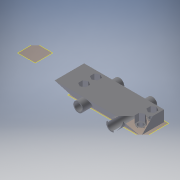
# Autodesk Inventor part: 23_Connection_Smartphone
Saved by Autodesk Inventor 2016 (Build 200138000, 138)
## iProperties
Created: 2016-10-24
Part Number: 23_Connection_Smartphone
Material: Generisch
Document SubType Name: Modeling
Designer: Bene
Density: 1 g/cm^3
Appearance: Vorgabe
Author: Bene
Autodesk Inventor part; units mm, degrees
ref_plane "YZ Plane" through (0, 0, 0) normal (1, 0, 0) x (0, 1, 0)
ref_plane "XZ Plane" through (0, 0, 0) normal (0, 1, 0) x (-1, 0, 0)
ref_plane "XY Plane" through (0, 0, 0) normal (0, 0, 1) x (1, 0, 0)
ref_plane "Arbeitsebene1" through (0, 0, 0) normal (0, 0, 1) x (1, 0, 0)
sketch "Skizze1" plane through (0, 0, 0) normal (0, 0, 1) x (1, 0, 0)
  circle A0 centre (-24, 5) radius 2.25 projected
  circle A1 centre (24, -5) radius 2.25 projected
  circle A2 centre (24, 5) radius 2.25 projected
  circle A3 centre (-24, -5) radius 2.25 projected
  line L0 (-29, 10) -> (-29, -10) projected
  line L1 (-29, -10) -> (29, -10) projected
  line L2 (29, -10) -> (29, 10) projected
  line L3 (29, 10) -> (-29, 10) projected
  ellipse E0 centre (-67.5, -3.1315) end of major axis (-59.5, -3.1315) minor radius 8 construction
  point P0 (0, 0)
  constraints: 1 other
ref_plane "Arbeitsebene2" through (-67.5, -3.1327, 9.2179) normal (0, -0.0022786, 0.9999974) x (0, -0.9999974, -0.0022786)
sketch "Skizze4" plane through (-67.5, -3.1327, 9.2179) normal (0, -0.0022786, 0.9999974) x (0, -0.9999974, -0.0022786)
  ellipse E0 centre (-0.5857, 0) end of major axis (-0.5857, -12.5) minor radius 12.4999 projected
  ellipse E1 centre (-8.1116, 43.5) end of major axis (-8.1116, 45.75) minor radius 2.25 construction
  ellipse E2 centre (1.8883, 91.5) end of major axis (1.8883, 93.75) minor radius 2.25 construction
  ellipse E3 centre (-8.1116, 91.5) end of major axis (-8.1116, 93.75) minor radius 2.25 construction
  ellipse E4 centre (1.8883, 43.5) end of major axis (1.8883, 45.75) minor radius 2.25 construction
  line L0 (-13.1116, 38.5) -> (6.8883, 38.5) construction
  line L1 (6.8883, 38.5) -> (6.8883, 96.5) construction
  line L2 (6.8883, 96.5) -> (-13.1116, 96.5) construction
  line L3 (-13.1116, 96.5) -> (-13.1116, 38.5) construction
  line L4 (11.9401, 96.5) -> (-13.1116, 96.5)
  line L5 (-13.1116, 96.5) -> (-13.1116, 38.5)
  line L6 (-13.1116, 38.5) -> (11.9401, 38.5)
  line L7 (11.9401, 38.5) -> (11.9401, 96.5)
  line L8 (11.9401, 96.5) -> (-13.1116, 38.5) construction
  line L9 (-13.1116, 96.5) -> (11.9401, 38.5) construction
  ellipse E5 centre (1.8883, 91.5) end of major axis (1.8883, 93.75) minor radius 2.25 projected
  ellipse E6 centre (-8.1116, 91.5) end of major axis (-8.1116, 93.75) minor radius 2.25 projected
  ellipse E7 centre (1.8883, 43.5) end of major axis (1.8883, 45.75) minor radius 2.25 projected
  ellipse E8 centre (-8.1116, 43.5) end of major axis (-8.1116, 45.75) minor radius 2.25 projected
  line L10 (11.9401, 38.5) -> (-13.1116, 38.5)
  line L11 (-13.1116, 38.5) -> (-13.1116, 28.5)
  line L12 (-13.1116, 28.5) -> (11.9401, 28.5)
  line L13 (11.9401, 28.5) -> (11.9401, 38.5)
  point P0 (-3.1117, 67.5)
  point P1 (-0.5857, 67.5)
  dimension "d1" = 0
  dimension "d22" = 10
  constraints: 20 end point, 4 parallel, 2 horizontal, 2 midpoint, 2 perpendicular, 9 other
  measures "d1" horizontal distance of point (-0.586, 0) point (-0.586, 67.5)
  measures "d22" distance of L11.end L10.end
loft "Erhebung1" add profiles "Skizze1", "Skizze4" contours A0 | A1 | A2 | A3 | L3 L2 L1 L0 / L7 L6 L5 L4 | L13 L12 L11 L6 | E5 | E6 | E7 | E8
sketch "Skizze5" plane through (-29, 10, 0) normal (0, 0.9999974, 0.0022786) x (1, 0, 0)
  line L0 (58, 0) -> (0, 0) projected
  line L1 (58, -9.2478) -> (-10, -9.2478) projected
  line L2 (58, 0) -> (58, -9.2478) projected
  circle A0 centre (43, -4.6239) radius 3.15
  circle A1 centre (15, -4.6239) radius 3.15
  line L3 (0, 0) -> (-10, -9.2478) projected
  point P0 (29, -0.0228)
  dimension "d8" = 6.3
  dimension "d9" = 6.3
  constraints: 2 centre point, 2 coincident
  measures "d8" diameter of A0
  measures "d9" diameter of A1
extrude "Extrusion1" cut sketch "Skizze5" against normal through all contours A0 | A1
sketch "Skizze6" plane through (-29, 10, 0) normal (0, 0.9999974, 0.0022786) x (1, 0, 0)
  circle A0 centre (43, -4.6239) radius 3.15 projected
  circle A1 centre (15, -4.6239) radius 3.15 projected
  line L0 (58, 0) -> (0, 0) projected
  line L1 (58, -9.2478) -> (-10, -9.2478) projected
  line L2 (58, 0) -> (58, -9.2478) projected
  circle A2 centre (43, -4.6239) radius 4.15
  circle A3 centre (15, -4.6239) radius 4.15
  line L3 (0, 0) -> (-10, -9.2478) projected
  point P0 (29, -0.0228)
  dimension "d12" = 1
  dimension "d13" = 1
  constraints: 2 centre point
  measures "d12" radial gap between concentric circles of A0 A2
  measures "d13" radial gap between concentric circles of A1 A3
sketch "Skizze7" plane through (-29, -15.0728, 9.1907) normal (0, -0.0022786, 0.9999974) x (1, 0, 0)
  ellipse E0 centre (5, 10.0518) end of major axis (7.25, 10.0518) minor radius 2.25 projected
  ellipse E1 centre (5, 20.0518) end of major axis (7.25, 20.0518) minor radius 2.25 projected
  ellipse E2 centre (53, 20.0518) end of major axis (55.25, 20.0518) minor radius 2.25 projected
  ellipse E3 centre (53, 10.0518) end of major axis (55.25, 10.0518) minor radius 2.25 projected
  point P0 (29, 15.0518)
  constraints: 4 other
extrude "Extrusion2" add sketch "Skizze6" along normal blind 5 and the other way blind 30 contours A2 | A3
extrude "Extrusion3" cut sketch "Skizze7" against normal through all
sketch "Skizze8" plane through (-29, -15.0728, 9.1907) normal (0, -0.0022786, 0.9999974) x (1, 0, 0)
  ellipse E0 centre (5, 10.0518) end of major axis (2.75, 10.0518) minor radius 2.25 projected
  ellipse E1 centre (5, 20.0518) end of major axis (2.75, 20.0518) minor radius 2.25 projected
  ellipse E2 centre (53, 20.0518) end of major axis (50.75, 20.0518) minor radius 2.25 projected
  ellipse E3 centre (53, 10.0518) end of major axis (50.75, 10.0518) minor radius 2.25 projected
  line L0 (1.8083, 8.2091) -> (1.8083, 11.8945)
  line L1 (1.8083, 11.8945) -> (5, 13.7373)
  line L2 (5, 13.7373) -> (8.1917, 11.8945)
  line L3 (8.1917, 11.8945) -> (8.1917, 8.2091)
  line L4 (8.1917, 8.2091) -> (5, 6.3663)
  line L5 (5, 6.3663) -> (1.8083, 8.2091)
  line L6 (0, 25.0518) -> (0, 0) projected
  line L7 (8.2124, 18.1971) -> (5, 16.3424)
  line L8 (5, 16.3424) -> (1.7876, 18.1971)
  line L9 (1.7876, 18.1971) -> (1.7876, 21.9065)
  line L10 (1.7876, 21.9065) -> (5, 23.7611)
  line L11 (5, 23.7611) -> (8.2124, 21.9065)
  line L12 (8.2124, 21.9065) -> (8.2124, 18.1971)
  line L13 (49.774, 18.1893) -> (49.774, 21.9143)
  line L14 (49.774, 21.9143) -> (53, 23.7768)
  line L15 (53, 23.7768) -> (56.226, 21.9143)
  line L16 (56.226, 21.9143) -> (56.226, 18.1893)
  line L17 (56.226, 18.1893) -> (53, 16.3268)
  line L18 (53, 16.3268) -> (49.774, 18.1893)
  line L19 (58, 0) -> (58, 25.0518) projected
  line L20 (49.7826, 8.1942) -> (49.7826, 11.9094)
  line L21 (49.7826, 11.9094) -> (53, 13.767)
  line L22 (53, 13.767) -> (56.2174, 11.9094)
  line L23 (56.2174, 11.9094) -> (56.2174, 8.1942)
  line L24 (56.2174, 8.1942) -> (53, 6.3366)
  line L25 (53, 6.3366) -> (49.7826, 8.1942)
  line L26 (-10, 25.0518) -> (-10, 0) projected
  point P0 (29, 15.0518)
  constraints: 48 end point, 5 parallel, 4 coincident, 56 other
extrude "Extrusion4" cut sketch "Skizze8" against normal blind 6
